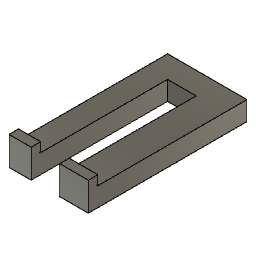
jig (Autodesk Fusion 360 design; units mm, degrees)
Autodesk Fusion 360 part; units mm, degrees
sketch "Sketch2" plane through (0, 0, 0) normal (0, 0, 1) x (1, 0, 0) in component "jig"
  line L0 (0, 0) -> (0, 160)
  line L1 (0, 160) -> (134, 160)
  line L2 (134, 160) -> (134, 0)
  line L3 (134, 0) -> (0, 0)
  line L4 (40, 160) -> (58, 160)
  line L5 (58, 160) -> (58, 60)
  line L6 (58, 60) -> (40, 60)
  line L7 (40, 60) -> (40, 160)
  line L8 (76, 0) -> (94, 0)
  line L9 (94, 0) -> (94, 80)
  line L10 (94, 80) -> (76, 80)
  line L11 (76, 80) -> (76, 0)
  line L12 (76, 80) -> (58, 80) construction
  line L13 (0, 160) -> (40, 160)
  line L14 (40, 160) -> (40, 166)
  line L15 (40, 166) -> (0, 166)
  line L16 (0, 166) -> (0, 160)
  line L17 (134, 160) -> (58, 160)
  line L18 (58, 160) -> (58, 166)
  line L19 (58, 166) -> (134, 166)
  line L20 (134, 166) -> (134, 160)
  line L21 (0, 0) -> (76, 0)
  line L22 (76, 0) -> (76, -6)
  line L23 (76, -6) -> (0, -6)
  line L24 (0, -6) -> (0, 0)
  line L25 (134, 0) -> (94, 0)
  line L26 (94, 0) -> (94, -6)
  line L27 (94, -6) -> (134, -6)
  line L28 (134, -6) -> (134, 0)
  dimension "d18" = 18
  dimension "d21" = 80
  dimension "d22" = 60
  dimension "d23" = 80
  dimension "d25" = 40
  dimension "d27" = 40
  dimension "d28" = 6
  dimension "d29" = 6
  constraint coincident L0.start L3.end
  constraint vertical L0
  constraint perpendicular L0 L1
  constraint perpendicular L1 L2
  constraint perpendicular L0 L3
  constraint horizontal L4
  constraint vertical L5
  constraint horizontal L6
  constraint vertical L7
  constraint coincident L1 L4.start
  constraint horizontal L8
  constraint vertical L9
  constraint horizontal L10
  constraint vertical L11
  constraint coincident L3 L8.start
  constraint equal L6 L10
  constraint coincident L11 L10.end
  constraint coincident L5 L12.end
  constraint perpendicular L5 L12
  constraint equal L6 L12
  constraint coincident L10.end L11.start
  constraint horizontal L13
  constraint vertical L14
  constraint horizontal L15
  constraint vertical L16
  constraint horizontal L17
  constraint vertical L18
  constraint horizontal L19
  constraint vertical L20
  constraint horizontal L21
  constraint vertical L22
  constraint horizontal L23
  constraint vertical L24
  constraint horizontal L25
  constraint vertical L26
  constraint horizontal L27
  constraint vertical L28
  constraint collinear L23 L27
  constraint collinear L15 L19
  constraint collinear L7 L14
  constraint collinear L5 L18
  constraint collinear L11 L22
  constraint collinear L9 L26
  measures "d18" distance of L5.end L6.end
  measures "d21" distance of L1 L10
  measures "d22" distance of L3 L6
  measures "d23" distance of L8.start L10.end
  measures "d25" distance of L0 L7
  measures "d27" distance of L2 L9
  measures "d28" distance of L0.end L15.end
  measures "d29" distance of L0.start L23.end
extrude "Extrude1" add sketch "Sketch2" along normal blind 12 contours L0 L1 L2 L3 L5 L6 L7 L9 L10 L11 L13 L17 L21 L25 in component "jig"
extrude "Extrude2" add sketch "Sketch2" along normal blind 18 contours L3 L21 L22 L23 L24 | L1 L13 L14 L15 L16 | L3 L25 L26 L27 L28 | L1 L17 L18 L19 L20 in component "jig"
sketch "Sketch3" plane through (0, 0, 0) normal (-1, 0, 0) x (0, -1, 0) in component "jig"
  line L0 (-166, 0) -> (6, 0)
  line L1 (6, 0) -> (6, 18)
  line L2 (6, 18) -> (0, 18)
  line L3 (0, 18) -> (0, 12)
  line L4 (0, 12) -> (-160, 12)
  line L5 (-160, 12) -> (-160, 18)
  line L6 (-160, 18) -> (-166, 18)
  line L7 (-166, 18) -> (-166, 0)
  line L8 (-160, 13) -> (-160.4879, 12.5121)
  line L9 (-160.2757, 12) -> (-160, 12)
  line L10 (-160, 13) -> (-160, 12)
  arc A0 (-160.4879, 12.5121) -> (-160.2757, 12) centre (-160.2757, 12.3) ccw
  line L11 (0, 12) -> (0.2757, 12)
  line L12 (0.4879, 12.5121) -> (0, 13)
  line L13 (0, 12) -> (0, 13)
  arc A1 (0.2757, 12) -> (0.4879, 12.5121) centre (0.2757, 12.3) ccw
  dimension "d34" = 1
  dimension "d35" = 0.3
  dimension "d36" = 45
  dimension "d37" = 1
  dimension "d38" = 45
  dimension "d39" = 0.3
  constraint coincident L5 L8.start
  constraint coincident L4.end L5.start
  constraint perpendicular L5 L9
  constraint tangent L8 A0
  constraint tangent L9 A0
  constraint coincident L3.end L4.start
  constraint perpendicular L3 L11
  constraint coincident L3 L12.end
  constraint tangent L11 A1
  constraint tangent L12 A1
  measures "d34" distance of L8.start L4.end
  measures "d35" radius of A0
  measures "d36" angle of L8 L10
  measures "d37" distance of L3.end L12.end
  measures "d38" angle of L12 L13
  measures "d39" radius of A1
extrude "Extrude3" cut sketch "Sketch3" against normal up to surface (134 mm away) contours L5 L8 L9 L10 A0 | L3 L11 L12 L13 A1 in component "jig"
box "BoxPrimitive1" cut length 30 width 50 height -100 placed x (0, 0, -1) y (1, 0, 0) z (0, -1, 0) at (62.0445, -6, 30) keep common part in component "jig"
component "jig" placed x (1, 0, 0) y (0, 1, 0) z (0, 0, 1) at (0, 0, 0)
equation "stockW = 200 mm"
equation "stockH = 120 mm"
equation "stockT = 18 mm"
equation "lipT = stockT / 3"
equation "lipH = lipT"
equation "jigT = 12 mm"
equation "stock2H = 160 mm"
equation "d18 = stockT"
equation "d21 = stock2H / 2"
equation "d22 = stockH / 2"
equation "d23 = stock2H / 2"
equation "baseMargin = 40 mm"
equation "d25 = baseMargin"
equation "d27 = baseMargin"
equation "d28 = lipT"
equation "d29 = lipT"
equation "d30 = jigT"
equation "d32 = jigT + lipT"
